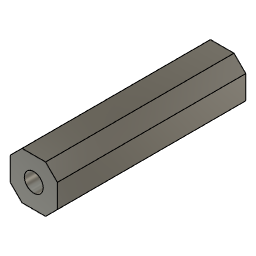
Collin_Straight Connector v1 v3 (Autodesk Fusion 360 design; units mm, degrees)
Autodesk Fusion 360 part; units mm, degrees
sketch "Sketch1" plane through (0, 0, 0) normal (0, 1, 0) x (1, 0, 0)
  line L0 (0, 0) -> (4, 0)
  line L1 (4, 0) -> (4, -4)
  line L2 (4, -4) -> (0, -4)
  line L3 (0, -4) -> (0, 0)
  circle A0 centre (2, -2) radius 0.8
  dimension "d1" = 4
  dimension "d2" = 4
  dimension "BORE" = 1.6
  dimension "d4" = 2
  dimension "d5" = 2
  constraint horizontal L0
  constraint vertical L1
  constraint horizontal L2
  constraint vertical L3
  constraint coincident L0.start L3.end
  measures "d1" distance of L0.end L1.end
  measures "d2" distance of L1.end L2.end
  measures "BORE" diameter of A0
  measures "d4" distance of L0 A0.centre
  measures "d5" distance of L1 A0.centre
extrude "Extrude1" add sketch "Sketch1" along normal blind 16
chamfer "Chamfer1" distance 1 angle 45 4 edges at (4, 8, 4) (0, 8, 4) (0, 8, 0) (4, 8, 0)
